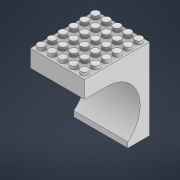
# Autodesk Inventor part: 110033226_ipt_19_大橋接通道路
Saved by Autodesk Inventor 2022 (Build 260153000, 153)
## iProperties
Created: 2022-06-23
Part Number: 110033226_ipt_19_大橋接通道路
Material: 一般
Document SubType Name: Modeling
Designer: User
Density: 1 g/cm^3
Appearance: 預設
Author: User
Autodesk Inventor part; units mm, degrees
ref_plane "YZ Plane" through (0, 0, 0) normal (1, 0, 0) x (0, 1, 0)
ref_plane "XZ Plane" through (0, 0, 0) normal (0, 1, 0) x (-1, 0, 0)
ref_plane "XY Plane" through (0, 0, 0) normal (0, 0, 1) x (1, 0, 0)
sketch "草圖1" plane through (0, 0, 0) normal (0, 1, 0) x (-1, 0, 0)
  line L0 (12.5, 12.5) -> (-12.5, 12.5)
  line L1 (-12.5, 12.5) -> (-12.5, -12.5)
  line L2 (-12.5, -12.5) -> (12.5, -12.5)
  line L3 (12.5, -12.5) -> (12.5, 12.5)
  circle A0 centre (10, 10) radius 1.7
  circle A1 centre (5, 10) radius 1.7
  circle A2 centre (0, 10) radius 1.7
  circle A3 centre (-5, 10) radius 1.7
  circle A4 centre (-10, 10) radius 1.7
  circle A5 centre (10, 5) radius 1.7
  circle A6 centre (5, 5) radius 1.7
  circle A7 centre (0, 5) radius 1.7
  circle A8 centre (-5, 5) radius 1.7
  circle A9 centre (-10, 5) radius 1.7
  circle A10 centre (10, 0) radius 1.7
  circle A11 centre (5, 0) radius 1.7
  circle A12 centre (0, 0) radius 1.7
  circle A13 centre (-5, 0) radius 1.7
  circle A14 centre (-10, 0) radius 1.7
  circle A15 centre (10, -5) radius 1.7
  circle A16 centre (5, -5) radius 1.7
  circle A17 centre (0, -5) radius 1.7
  circle A18 centre (-5, -5) radius 1.7
  circle A19 centre (-10, -5) radius 1.7
  circle A20 centre (10, -10) radius 1.7
  circle A21 centre (5, -10) radius 1.7
  circle A22 centre (0, -10) radius 1.7
  circle A23 centre (-5, -10) radius 1.7
  circle A24 centre (-10, -10) radius 1.7
  point P0 (0, 0)
  point P1 (12.5, 0)
  point P2 (0, -12.5)
  dimension "d0" = 25
  dimension "d1" = 25
  dimension "d10" = 3.4
  dimension "d11" = 2.5
  dimension "d12" = 2.5
  dimension "d15" = 5
  dimension "d18" = 5
  constraints: 25 centre point, 8 end point, 2 horizontal, 2 midpoint, 2 parallel, 1 horizontal alignment, 1 perpendicular, 1 vertical, 1 vertical alignment, 48 other
  measures "d0" distance of L2.end L1.end
  measures "d1" distance of L1.end L0.end
  measures "d10" diameter of A0
  measures "d11" distance from line of L0 A0.centre
  measures "d12" distance from line of L3 A0.centre
  measures "d15" distance of A0.centre A1.centre
  measures "d18" distance of A0.centre A5.centre
sketch "草圖2" plane through (0, 0, 0) normal (1, 0, 0) x (0, 1, 0)
  line L0 (0, 12.5) -> (0, -12.5) projected
  line L1 (0, -12.5) -> (35, -12.5)
  line L2 (35, -12.5) -> (35, 12.5)
  line L3 (35, 12.5) -> (27, 12.5)
  line L4 (27, 12.5) -> (27, 7.5)
  line L5 (0, -12.5) -> (0, -2.5)
  arc A0 (0, -2.5) -> (27, 7.5) centre (11.8134, 7.0537) ccw
  point P0 (0, 0)
  dimension "d2" = 35
  dimension "d3" = 8
  dimension "d4" = 5
  dimension "d5" = 10
  dimension "d6" = 25
  dimension "d7" = 15.1931
  constraints: 10 end point, 3 perpendicular, 2 point on circle, 1 centre point, 1 horizontal, 1 point on line
  measures "d2" distance of L0.end L1.end
  measures "d3" distance of L2.end L3.end
  measures "d4" distance of L3.end L4.end
  measures "d5" distance of L0.end L5.end
  measures "d6" distance of L1.end L2.end
  measures "d7" radius of A0
extrude "擠出1" add sketch "草圖2" along normal mid plane 25
sketch "草圖3" plane through (-12.5, 35, 12.5) normal (0, 1, 0) x (1, 0, 0)
  circle A0 centre (22.5, 22.5) radius 1.7 projected
  point P0 (12.5, 12.5)
extrude "擠出3" add sketch "草圖3" along normal blind 1.5
pattern_linear "矩形陣列1" count 5 spacing 5 along (-1, 0, 0) count 6 spacing 5 along (0, 0, 1) of "擠出3"
sketch "草圖4" plane through (-12.5, 27, 12.5) normal (0, 0, 1) x (1, 0, 0)
  line L0 (0, 0) -> (25, 0) projected
  line L1 (25, 8) -> (25, 0) projected
  line L2 (0, 8) -> (25, 8) projected
  line L3 (0, 0) -> (0, 8) projected
  line L4 (0, 8) -> (25, 8)
  line L5 (25, 8) -> (25, 0)
  line L6 (25, 0) -> (0, 0)
  line L7 (0, 0) -> (0, 8)
  point P0 (12.5, -27)
  constraints: 8 end point, 2 parallel, 1 horizontal, 1 perpendicular
extrude "擠出4" add sketch "草圖4" along normal blind 5
sketch "草圖5" plane through (-12.5, 0, -12.5) normal (0, -1, 0) x (1, 0, 0)
  line L0 (0, 10) -> (25, 10) projected
  line L1 (25, 10) -> (25, 0) projected
  line L2 (0, 0) -> (25, 0) projected
  line L3 (0, 0) -> (0, 10) projected
  point P0 (12.5, 12.5)
extrude "擠出5" add sketch "草圖5" along normal blind 2.5
sketch "草圖6" plane through (-12.5, -2.5, -12.5) normal (0, -1, 0) x (1, 0, 0)
  circle A0 centre (22.5, 7.5) radius 1.7 projected
  circle A1 centre (22.5, 2.5) radius 1.7 projected
  circle A2 centre (17.5, 7.5) radius 1.7 projected
  line L0 (25, 0) -> (25, 10) projected
  line L1 (25, 10) -> (0, 10) projected
  line L2 (0, 10) -> (0, 0) projected
  line L3 (0, 0) -> (25, 0) projected
  circle A3 centre (12.5, 7.5) radius 1.7 projected
  circle A4 centre (12.5, 2.5) radius 1.7 projected
  circle A5 centre (17.5, 2.5) radius 1.7 projected
  circle A6 centre (7.5, 7.5) radius 1.7 projected
  circle A7 centre (7.5, 2.5) radius 1.7 projected
  circle A8 centre (2.5, 7.5) radius 1.7 projected
  circle A9 centre (2.5, 2.5) radius 1.7 projected
  point P0 (12.5, 12.5)
extrude "擠出6" cut sketch "草圖6" against normal blind 1.5 contours A0 | A1 | A2 | A3 | A4 | A5 | A6 | A7 | A8 | A9
